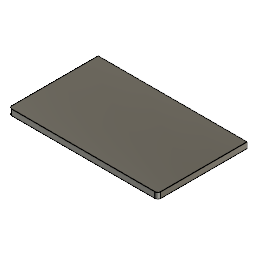
StanleySeparator (Autodesk Fusion 360 design; units mm, degrees)
Autodesk Fusion 360 part; units mm, degrees
sketch "Sketch1" plane through (0, 0, 0) normal (0, 0, 1) x (1, 0, 0)
  line L0 (24, -15) -> (-24, -15)
  line L1 (-25, -14) -> (-25, 15)
  line L2 (-25, 15) -> (25, 15)
  line L3 (25, 15) -> (25, -14)
  line L4 (25.9629, -15.5777) -> (-25, 15) construction
  line L5 (-25, -15) -> (25, 15) construction
  arc A0 (-25, -14) -> (-24, -15) centre (-24, -14) ccw
  arc A1 (24, -15) -> (25, -14) centre (24, -14) ccw
  dimension "d2" = 30
  dimension "d3" = 1
  dimension "d4" = 1
  dimension "d7" = 25
  dimension "d8" = 25
  measures "d2" distance of L5.start L1.end
  measures "d3" radius of A0
  measures "d4" radius of A1
  measures "d7" distance of origin L1
  measures "d8" distance of origin L3
extrude "Extrude1" add sketch "Sketch1" along normal blind 2
named bodies: "Separator"
